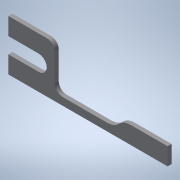
# Autodesk Inventor part: HarveyHeadplate_LargerCenter_FrontAndSideCutout_WiderTeeth_Ver3
Saved by Autodesk Inventor 2022 (Build 260153000, 153)
## iProperties
Created: 2011-10-05
Part Number: HarveyHeadplate_LargerCenter_FrontAndSideCutout_WiderTeeth_Ver3
Material: Generic
Document SubType Name: Modeling
Designer: charvey
Density: 1 g/cm^3
Appearance: Default
Author: charvey
Autodesk Inventor part; units mm, degrees
ref_plane "YZ Plane" through (0, 0, 0) normal (1, 0, 0) x (0, 1, 0)
ref_plane "XZ Plane" through (0, 0, 0) normal (0, 1, 0) x (-1, 0, 0)
ref_plane "XY Plane" through (0, 0, 0) normal (0, 0, 1) x (1, 0, 0)
sketch "Sketch1" plane through (0, 0, 0) normal (0, 0, 1) x (1, 0, 0)
  line L0 (-15.24, 5.08) -> (15.24, 5.08)
  line L1 (15.24, 5.08) -> (15.24, -5.08)
  line L2 (15.24, -5.08) -> (-15.24, -5.08)
  line L3 (-15.24, -5.08) -> (-15.24, 5.08)
  point P0 (0, 0)
  point P1 (0, 5.08)
  point P2 (-15.24, 0)
  dimension "d0" = 30.48
  dimension "d1" = 10.16
  constraints: 8 end point, 2 midpoint, 2 parallel, 1 horizontal, 1 horizontal alignment, 1 perpendicular, 1 vertical alignment
  measures "d0" distance between parallel lines of L1 L3
  measures "d1" distance between parallel lines of L2 L0
extrude "Extrusion1" add sketch "Sketch1" along normal blind 0.8128
sketch "Sketch2" plane through (0, 0, 0.8128) normal (0, 0, 1) x (1, 0, 0)
  line L0 (15.24, 5.08) -> (15.24, -5.08) projected
  line L1 (-15.24, 5.08) -> (15.24, 5.08) projected
  line L2 (-15.24, -5.08) -> (-15.24, 5.08) projected
  line L3 (15.24, -5.08) -> (-15.24, -5.08) projected
  line L4 (-4.3525, 3.556) -> (2.3785, 3.556)
  line L5 (-4.3525, -3.556) -> (2.3785, -3.556)
  line L6 (-5.94, 1.9685) -> (-5.94, -1.9685)
  line L7 (3.966, 1.9685) -> (3.966, -1.9685)
  arc A0 (-4.3525, 3.556) -> (-5.94, 1.9685) centre (-4.3525, 1.9685) ccw
  arc A1 (-5.94, -1.9685) -> (-4.3525, -3.556) centre (-4.3525, -1.9685) ccw
  arc A2 (2.3785, -3.556) -> (3.966, -1.9685) centre (2.3785, -1.9685) ccw
  arc A3 (3.966, 1.9685) -> (2.3785, 3.556) centre (2.3785, 1.9685) ccw
  point P0 (-0.987, 3.556)
  point P1 (-0.987, -3.556)
  point P2 (-5.94, 0)
  point P3 (3.966, 0)
  dimension "d5" = 6.731
  dimension "d6" = 6.731
  dimension "d7" = 3.937
  dimension "d8" = 3.937
  dimension "d13" = 1.5875
  dimension "d14" = 1.5875
  dimension "d15" = 1.5875
  dimension "d16" = 1.5875
  dimension "d38" = 9.3
  constraints: 8 end point, 8 point on circle, 4 centre point, 4 midpoint, 3 parallel, 1 perpendicular
  measures "d5" distance of L4.end L4.start
  measures "d6" distance of L5.end L5.start
  measures "d7" distance of L6.end L6.start
  measures "d8" distance of L7.end L7.start
  measures "d13" radius of A0
  measures "d14" radius of A1
  measures "d15" radius of A2
  measures "d16" radius of A3
  measures "d38" distance between parallel lines of L2 L6
extrude "Extrusion2" cut sketch "Sketch2" against normal blind 25.4 contours L4 A3 L7 A2 L5 A1 L6 A0
sketch "Sketch3" plane through (0, 0, 0.8128) normal (0, 0, 1) x (1, 0, 0)
  arc A0 (-4.3525, 3.556) -> (-5.94, 1.9685) centre (-4.3525, 1.9685) ccw projected
  line L0 (-4.3525, 3.556) -> (2.3785, 3.556) projected
  arc A1 (3.966, 1.9685) -> (2.3785, 3.556) centre (2.3785, 1.9685) ccw projected
  line L1 (3.966, 1.9685) -> (3.966, -1.9685) projected
  arc A2 (2.3785, -3.556) -> (3.966, -1.9685) centre (2.3785, -1.9685) ccw projected
  line L2 (2.3785, -3.556) -> (-4.3525, -3.556) projected
  arc A3 (-5.94, -1.9685) -> (-4.3525, -3.556) centre (-4.3525, -1.9685) ccw projected
  line L3 (-5.94, -1.9685) -> (-5.94, 1.9685) projected
  line L4 (15.24, 5.08) -> (15.24, -5.08) projected
  line L5 (-15.24, 5.08) -> (15.24, 5.08) projected
  line L6 (-15.24, -5.08) -> (-15.24, 5.08) projected
  line L7 (15.24, -5.08) -> (-15.24, -5.08) projected
  line L8 (-15.24, 1.5875) -> (-9.13, 1.5875)
  line L9 (-15.24, -1.5875) -> (-9.13, -1.5875)
  arc A4 (-9.13, -1.5875) -> (-9.13, 1.5875) centre (-9.13, 0) ccw
  point P0 (0, 0)
  dimension "d20" = 3.4925
  dimension "d21" = 6.11
  dimension "d22" = 3.175
  dimension "d24" = 1.5875
  constraints: 4 end point, 2 parallel, 2 point on circle, 2 point on line, 1 centre point
  measures "d20" distance between parallel lines of L8 L5
  measures "d21" distance of L9.start L9.end
  measures "d22" distance between parallel lines of L8 L9
  measures "d24" radius of A4
extrude "Extrusion3" cut sketch "Sketch3" against normal blind 25.4 contours L8 A4 L9 L6
mirror "Mirror1" about plane through (0, 0, 0) normal (1, 0, 0) of "Extrusion3"
sketch "Sketch5" plane through (0, 0, 0.8128) normal (0, 0, 1) x (1, 0, 0)
  line L0 (3.966, 1.9685) -> (3.966, -1.9685) construction
  line L1 (-5.94, -1.9685) -> (3.966, -1.9685)
  line L2 (3.966, -1.9685) -> (3.966, 7.0011)
  line L3 (3.966, 7.0011) -> (-5.94, 7.0011)
  line L4 (-5.94, 7.0011) -> (-5.94, -1.9685)
  point P0 (0, 0)
  constraints: 8 end point, 2 parallel, 1 horizontal, 1 perpendicular, 1 point on line
extrude "Extrusion5" cut sketch "Sketch5" against normal through all
fillet "Fillet1" radius 1.524 2 edges at (-5.94, 5.08, 0.4064) (3.966, 5.08, 0.4064)
sketch "Sketch7" plane through (0, 0, 0.8128) normal (0, 0, 1) x (1, 0, 0)
  line L0 (9.13, -1.5875) -> (15.24, -1.5875) construction
  line L1 (15.24, -1.5875) -> (3.966, -1.5875)
  line L2 (3.966, -1.5875) -> (3.966, 5.08)
  line L3 (3.966, 5.08) -> (15.24, 5.08)
  line L4 (15.24, 5.08) -> (15.24, -1.5875)
  line L5 (3.966, 3.556) -> (3.966, -1.9685) projected
  point P0 (0, 0)
  constraints: 8 end point, 2 parallel, 1 collinear, 1 horizontal, 1 perpendicular
extrude "Extrusion6" cut sketch "Sketch7" against normal through all
sketch "Sketch8" plane through (0, 0, 0.8128) normal (0, 0, 1) x (1, 0, 0)
  line L0 (3.966, -1.5875) -> (15.24, -1.5875) projected
  arc A0 (2.3785, -3.556) -> (3.966, -1.9685) centre (2.3785, -1.9685) ccw projected
  line L1 (7.62, -1.5875) -> (2.3785, -1.5875)
  line L2 (2.3785, -1.5875) -> (2.3785, -3.556)
  line L3 (2.3785, -3.556) -> (7.62, -3.556)
  line L4 (7.62, -3.556) -> (7.62, -1.5875)
  line L5 (15.24, -1.5875) -> (15.24, -5.08) projected
  point P0 (0, 0)
  dimension "d34" = 7.62
  constraints: 8 end point, 2 parallel, 1 horizontal, 1 perpendicular, 1 point on line
  measures "d34" distance between parallel lines of L5 L4
extrude "Extrusion7" cut sketch "Sketch8" against normal through all
fillet "Fillet2" radius 3.175 2 edges at (7.62, -3.556, 0.4064) (7.62, -1.5875, 0.4064)
sketch "Sketch9" plane through (15.24, -5.08, 0.8128) normal (1, 0, 0) x (0, 0, -1)
  line L0 (0.8128, 3.4925) -> (0, 3.4925) projected
  line L1 (0, 3.4925) -> (0, 0) projected
  line L2 (0.8128, 0) -> (0, 0) projected
  line L3 (0.8128, 3.4925) -> (0.8128, 0) projected
  point P0 (0.8128, 5.08)
extrude "Extrusion8" add sketch "Sketch9" along normal blind 1.5
body "Solid1"
